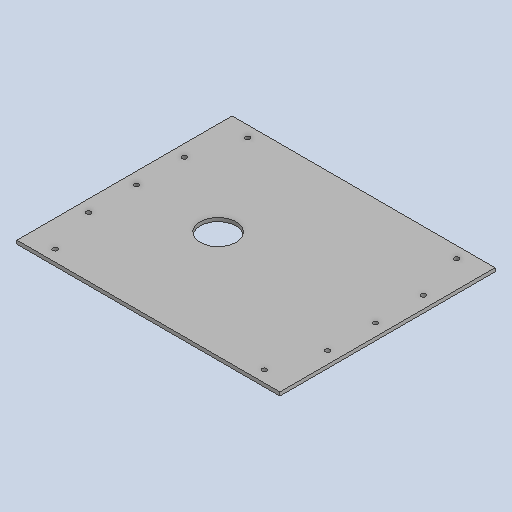
# Autodesk Inventor part: 000.003 - cap
Saved by Autodesk Inventor 2022 (Build 260153000, 153)
## iProperties
Created: 2021-06-26
Part Number: 000.003 - cap
Material: Типовые
Document SubType Name: Modeling
Designer: Петров Иван
Mass: 116.302 g
Surface Area: 805.947 cm^2
Volume: 116.302 cm^3
Density: 1 g/cm^3
Appearance: По умолчанию
Author: Петров Иван
Autodesk Inventor part; units mm, degrees
ref_plane "YZ Plane" through (0, 0, 0) normal (1, 0, 0) x (0, 1, 0)
ref_plane "XZ Plane" through (0, 0, 0) normal (0, 1, 0) x (-1, 0, 0)
ref_plane "XY Plane" through (0, 0, 0) normal (0, 0, 1) x (1, 0, 0)
sketch "Эскиз1" plane through (0, 0, 0) normal (0, 1, 0) x (-1, 0, 0)
  line L0 (-110, 90) -> (110, 90)
  line L1 (110, 90) -> (110, -90)
  line L2 (110, -90) -> (-110, -90)
  line L3 (-110, -90) -> (-110, 90)
  line L4 (-110, 90) -> (110, -90) construction
  line L5 (110, 90) -> (-110, -90) construction
  point P0 (0, 0)
  dimension "d0" = 220
  dimension "d1" = 180
  constraints: 12 end point, 2 midpoint, 2 parallel, 1 horizontal, 1 perpendicular
  measures "d0" distance of L1.end L2.end
  measures "d1" distance of L0.end L1.end
extrude "Выдавливание1" add sketch "Эскиз1" along normal blind 3
sketch "Эскиз2" plane through (0, 0, 0) normal (0, -1, 0) x (1, 0, 0)
  circle A0 centre (99.9996, -40) radius 2 projected
  circle A1 centre (99.9996, 0) radius 2 projected
  circle A2 centre (99.9996, 40) radius 2 projected
  circle A3 centre (-99.9997, 0) radius 2 projected
  circle A4 centre (-99.9997, -40) radius 2 projected
  circle A5 centre (-99.9997, 40) radius 2 projected
  point P0 (0, 0)
extrude "Выдавливание2" cut sketch "Эскиз2" against normal blind 3
sketch "Эскиз3" plane through (0, 3, 0) normal (0, 1, 0) x (1, 0, 0)
  circle A0 centre (87.4999, 80.5) radius 2 projected
  circle A1 centre (-87.5001, 80.5) radius 2 projected
  circle A2 centre (-87.5001, -80.5) radius 2 projected
  circle A3 centre (87.4999, -80.5) radius 2 projected
  point P0 (0, 0)
extrude "Выдавливание3" cut sketch "Эскиз3" against normal blind 10
sketch "Эскиз4" plane through (0, 3, 0) normal (0, 1, 0) x (1, 0, 0)
  circle A0 centre (-31.6806, 0) radius 15 projected
  point P0 (0, 0)
extrude "Выдавливание4" cut sketch "Эскиз4" against normal blind 10
